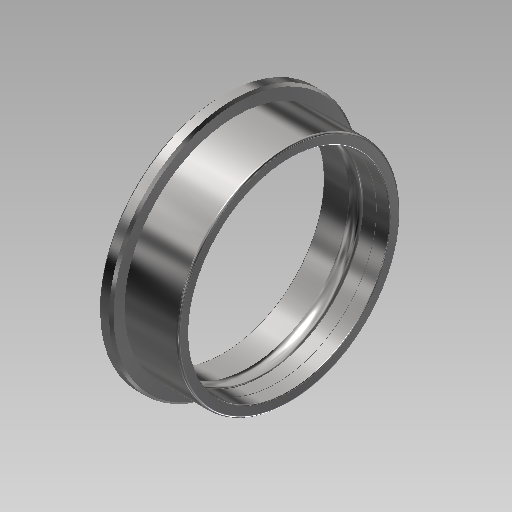
# Autodesk Inventor part: LF-1060ZZ_or
Saved by Autodesk Inventor 2021 (Build 250183000, 183)
## iProperties
Created: 2019-09-04
Part Number: LF-1060ZZ_or
Material: 鋼、炭素鋼
Catalog Web Link: www.cadenas.de
Description: Radial Flanged Ball Bearings (RF-Series/LF series) Metric ST or-Radial Flanged Ball Bearings (RF-Series/LF series) Metric Shielded Type
Vendor: NMB
Document SubType Name: Modeling
Designer: psadmin
Manufacturer: NMB
Mass: 0.427301 g
Surface Area: 2.45882 cm^2
Volume: 0.0544332 cm^3
Density: 7.85 g/cm^3
Appearance: 半つや出し
Category: PARTsolutions
Company: NMB
PSOL_IDENT_0: {$CADENAS_DATA\23d-libs\nmb\pbbp\radial_flanged_ball_bearings\rfbb_rflfs_m\rflf_shielded_or.prj},223
PSOL_IDENT_1: {VTYP=3D},{NB=LF-1060ZZ_or},{LINA=LF-1060ZZ_or},{NN=Radial Flanged Ball Bearings (RF-Series/LF seri
PSOL_IDENT_2: es) Metric ST or},{DATE=11.11.2013 05:13:45},{GEOMDATE=24.10.2013 13:34:00},{VERSION=},{LINEID=1200}
PSOL_IDENT_3: ,{WBVAR=},{WBNUMERIC=}  {NB=LF-1060ZZ_or},{LINA=LF-1060ZZ_or},{KT=DUMMY},{IDNR=},{PN=LF-1060ZZ},{SHL
PSOL_IDENT_4: D=shielded},{FLANG=flanged},{SD=6.000},{D=10.000},{B=3.000},{SR=0.10},{BCZ=9},{DW=1.1906},{LI=6.95},
PSOL_IDENT_5: {LO=9.04},{D1=11.200},{C1=0.60},{D2=0.0},{C2=0.00},{COR=194},{CR=1029},{PCD=8.000},{U=9.191},{W=6.80
PSOL_IDENT_6: 9},{Y=0.595},{Z=0.595},{AA=9.072},{AC=0.60},{AD=0.000},{AF=0.00},{AQ=0.20},{AH=9.24},{AI=7.15},{AJ=0
PSOL_IDENT_7: .40}
NN: Radial Flanged Ball Bearings (RF-Series/LF series) Metric ST or
NT: Radial Flanged Ball Bearings (RF-Series/LF series) Metric Shielded Type
NB: LF-1060ZZ_or
NBSYN: $PN._or
LINA: LF-1060ZZ_or
PN: LF-1060ZZ
SHLD: shielded
FLANG: flanged
SD: 6
D: 10
B: 3
SR: 0.1
BCZ: 9
DW: 1.1906
LI: 6.95
LO: 9.04
D1: 11.2
C1: 0.6
D2: 0
C2: 0
COR: 194
CR: 1029
PCD: 8
U: 9.191
W: 6.809
Y: 0.595
Z: 0.595
AA: 9.072
AC: 0.6
AD: 0
AF: 0
AQ: 0.2
AH: 9.24
AI: 7.15
AJ: 0.4
SUPPLIER: NMB
ARTICLENO: LF-1060ZZ_or
BOMINFO: LF-1060ZZ_or
CREATOR: CADENAS GmbH
Title: LF-1060ZZ_or
Author: Cadenas PARTsolutions
Comments: Radial Flanged Ball Bearings (RF-Series/LF series) Metric Shielded Type
Autodesk Inventor part; units mm, degrees
sketch "Sketch_3" plane through (0, 0, 0) normal (0, 0, 1) x (1, 0, 0)
  line L0 (2.9, 0) -> (0, 0)
  line L1 (0, 5.5) -> (0, 4.57)
  arc A0 (0, 4.57) -> (0.05, 4.52) centre (0.05, 4.57) ccw
  line L2 (0.05, 4.52) -> (0.605, 4.52)
  line L3 (0.605, 4.52) -> (0.605, 4.5001)
  line L4 (0.605, 4.5001) -> (1.177, 4.5001)
  arc A1 (1.823, 4.5001) -> (1.177, 4.5001) centre (1.5, 4) ccw
  line L5 (1.823, 4.5001) -> (2.4, 4.5001)
  line L6 (2.4, 4.5001) -> (2.4, 4.52)
  line L7 (2.4, 4.52) -> (2.95, 4.52)
  arc A2 (2.95, 4.52) -> (3, 4.57) centre (2.95, 4.57) ccw
  line L8 (3, 4.57) -> (3, 4.9)
  arc A3 (3, 4.9) -> (2.9, 5) centre (2.9, 4.9) ccw
  line L9 (2.9, 5) -> (0.6, 5)
  line L10 (0.6, 5) -> (0.6, 5.5)
  line L11 (0.6, 5.5) -> (0.5, 5.6)
  line L12 (0.5, 5.6) -> (0.1, 5.6)
  line L13 (0.1, 5.6) -> (0, 5.5)
  constraints: 28 end point, 8 point on circle, 4 centre point
revolve "Revolution1" add sketch "Sketch_3" angle 360 about axis through (2.9, 0, 0) along (1, 0, 0)
ref_plane "1_XY" through (1.5, 0, 0) normal (1, 0, 0) x (0, 0, -1)
ref_plane "1_YZ" through (1.5, 0, 0) normal (0, 0, -1) x (0, 1, 0)
ref_plane "1_ZX" through (1.5, 0, 0) normal (0, 1, 0) x (1, 0, 0)
body "Solid1"
